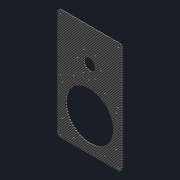
# Autodesk Inventor part: carbonplate2
Saved by Autodesk Inventor 2022 (Build 260153000, 153)
## iProperties
Created: 2021-09-16
Part Number: carbonplate2
Material: CFRP
Document SubType Name: Sheet Metal
Designer: Yuta Kage
Density: 1.43 g/cm^3
Sheet Metal Rule: Default_mm
Appearance: カーボンファイバー
Author: Yuta Kage
Autodesk Inventor part; units mm, degrees
ref_plane "YZ Plane" through (0, 0, 0) normal (1, 0, 0) x (0, 1, 0)
ref_plane "XZ Plane" through (0, 0, 0) normal (0, 1, 0) x (-1, 0, 0)
ref_plane "XY Plane" through (0, 0, 0) normal (0, 0, 1) x (1, 0, 0)
sketch "スケッチ1" plane through (0, 0, 0) normal (0, 0, 1) x (1, 0, 0)
  line L0 (-55, -95) -> (55, -95)
  line L1 (55, -95) -> (55, 95)
  line L2 (55, 95) -> (-55, 95)
  line L3 (-55, 95) -> (-55, -95)
  line L4 (-55, -95) -> (55, 95) construction
  line L5 (55, -95) -> (-55, 95) construction
  circle A0 centre (0, 40) radius 6.5
  line L6 (0, 40) -> (-55, 95)
  point P0 (0, 0)
  dimension "d0" = 110
  dimension "d39" = 45
  measures "d0" distance of L1.end L2.end
  measures "d39" angle of L2 L6
extrude "プレート1" add sketch "スケッチ1" along normal blind 2 contours L3 L2 L1 L0 | A0
sketch "スケッチ2" plane through (0, 0, 2) normal (0, 0, 1) x (1, 0, 0)
  circle A0 centre (0, -40) radius 12.5
  point P0 (0, 0)
  point P1 (0, -27.5)
  point P2 (-12.5, -40)
  point P3 (0, -52.5)
  point P4 (12.5, -40)
  dimension "d8" = 25
  dimension "d11" = 360
  constraints: 2 vertical alignment, 7 other
hole "穴1" at (0, -27.5, 2) at (-12.5, -40, 2) at (0, -52.5, 2) at (12.5, -40, 2) direction (0, 0, -1) diameter 3.2 end through all clearance for "Socket Head Cap Screw" size "M3" standard "Ansi Metric M Profile"
sketch "スケッチ3" plane through (0, 0, 2) normal (0, 0, 1) x (1, 0, 0)
  circle A0 centre (0, 38.4) radius 10
  point P0 (0, 0)
  dimension "d22" = 20
  dimension "d58" = 38.4
  constraints: 1 centre point, 1 vertical alignment
  measures "d22" diameter of A0
  measures "d58" distance of point (0, 0) A0.centre
extrude "押し出し1" cut sketch "スケッチ3" against normal blind 10
sketch "スケッチ4" plane through (0, 0, 2) normal (0, 0, 1) x (1, 0, 0)
  line L0 (-55, 95) -> (55, 95) projected
  line L1 (-55, -95) -> (-55, 95) projected
  line L2 (55, 95) -> (55, -95) projected
  line L3 (55, -95) -> (-55, -95) projected
  line L4 (50, 90) -> (-50, 90)
  line L5 (-50, 90) -> (-50, -90)
  line L6 (-50, -90) -> (50, -90)
  line L7 (50, -90) -> (50, 90)
  point P0 (0, 0)
  point P1 (-50, 0)
  point P2 (50, 0)
  dimension "d25" = 5
  constraints: 8 end point, 2 midpoint, 3 other
  measures "d25" distance between parallel lines of L0 L4
hole "穴2" at (-50, 90, 2) at (50, 90, 2) at (50, -90, 2) at (-50, -90, 2) at (50, 0, 2) at (-50, 0, 2) direction (0, 0, -1) diameter 4.3 end through all clearance for "Socket Head Cap Screw" size "M4" standard "Ansi Metric M Profile"
fillet "コーナーR1" radius 5 4 edges at (55, 95, 1) (-55, 95, 1) (-55, -95, 1) (55, -95, 1)
sketch "スケッチ5" plane through (0, 0, 2) normal (0, 0, 1) x (1, 0, 0)
  circle A0 centre (0, -38.4) radius 41
  point P0 (0, 0)
  dimension "d35" = 82
  dimension "d59" = 38.4
  constraints: 1 centre point
  measures "d35" diameter of A0
  measures "d59" distance of point (0, 0) A0.centre
extrude "押し出し2" cut sketch "スケッチ5" against normal blind 10
sketch "スケッチ6" plane through (0, 0, 2) normal (0, 0, 1) x (1, 0, 0)
  circle A0 centre (0, -38.4) radius 41 projected
  circle A1 centre (0, -38.4) radius 53.5
  circle A2 centre (0, 38.4) radius 10 projected
  circle A3 centre (0, 38.4) radius 20
  point P0 (0, 0)
  point P1 (-46.3324, -65.15)
  point P2 (-26.75, -84.7324)
  point P3 (0, -91.9)
  point P4 (26.75, -84.7324)
  point P5 (46.3324, -65.15)
  point P6 (53.5, -38.4)
  point P7 (46.3324, -11.65)
  point P8 (26.75, 7.9324)
  point P9 (0, 15.1)
  point P10 (-26.75, 7.9324)
  point P11 (-46.3324, -11.65)
  point P12 (-53.5, -38.4)
  point P13 (-10, 55.7205)
  point P14 (-20, 38.4)
  point P15 (-10, 21.0795)
  point P16 (10, 21.0795)
  point P17 (20, 38.4)
  point P18 (10, 55.7205)
  dimension "d40" = 107
  dimension "d52" = 40
  dimension "d43" = 360
  dimension "d55" = 360
  dimension "d57" = 0
  constraints: 2 coincident, 1 horizontal alignment, 26 other
  measures "d57" vertical distance of point (-10, 21.079) point (10, 21.079)
hole "穴3" at (-26.75, -84.7324, 2) at (-46.3324, -65.15, 2) at (-46.3324, -11.65, 2) at (-26.75, 7.9324, 2) at (26.75, 7.9324, 2) at (46.3324, -11.65, 2) at (46.3324, -65.15, 2) at (26.75, -84.7324, 2) at (10, 55.7205, 2) at (20, 38.4, 2) at (-20, 38.4, 2) at (-10, 55.7205, 2) at (0, 15.1, 2) at (10, 21.0795, 2) at (-10, 21.0795, 2) direction (0, 0, -1) diameter 3.2 end through all clearance for "Socket Head Cap Screw" size "M3" standard "Ansi Metric M Profile"
equation "\"d20\" = Thickness"
equation "\"d50\" = Thickness"
equation "\"d2\" = Thickness"
equation "\"BendRadius\" = Thickness"
equation "\"BendReliefWidth\" = Thickness"
equation "\"BendReliefDepth\" = 0.5 * Thickness"
equation "\"CornerReliefSize\" = 4 * Thickness"
equation "\"MinimumRemnant\" = 2 * Thickness"
equation "\"TransitionRadius\" = BendRadius"
equation "\"JacobiRadiusSize\" = BendRadius"
equation "\"GapSize\" = Thickness"
equation "\"Thickness\" = 2"
